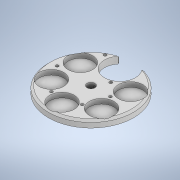
# Autodesk Inventor part: carousel_print
Saved by Autodesk Inventor 2021 (Build 250183000, 183)
## iProperties
Created: 2024-02-22
Part Number: carousel_print
Material: Generic
Document SubType Name: Modeling
Designer: Sebastián
Density: 1 g/cm^3
Appearance: Default
Author: Sebastián
Autodesk Inventor part; units mm, degrees
ref_plane "YZ Plane" through (0, 0, 0) normal (1, 0, 0) x (0, 1, 0)
ref_plane "XZ Plane" through (0, 0, 0) normal (0, 1, 0) x (-1, 0, 0)
ref_plane "XY Plane" through (0, 0, 0) normal (0, 0, 1) x (1, 0, 0)
sketch "Sketch1" plane through (0, 0, 0) normal (0, 1, 0) x (-1, 0, 0)
  circle A0 centre (0, 0) radius 44 construction
  circle A1 centre (0, 0) radius 4.1
  line L0 (0, -30) -> (-25.9808, -15) construction
  line L1 (-25.9808, -15) -> (-25.9808, 15) construction
  line L2 (-25.9808, 15) -> (0, 30) construction
  line L3 (0, 30) -> (25.9808, 15) construction
  line L4 (25.9808, 15) -> (25.9808, -15) construction
  line L5 (25.9808, -15) -> (0, -30) construction
  circle A2 centre (0, -30) radius 12.7 construction
  circle A3 centre (0, -30) radius 16 construction
  circle A4 centre (25.9808, -15) radius 12.7 construction
  arc A5 (9.3274, -43) -> (-9.3274, -43) centre (0, -30) ccw construction
  arc A6 (9.3274, -43) -> (-9.3274, -43) centre (0, 0) ccw
  line L6 (0, -64) -> (0, 62) projected
  arc A7 (9.3274, -43) -> (-9.3274, -43) centre (0, -30) ccw
  dimension "d0" = 88
  dimension "d4" = 32
  dimension "d1" = 8.2
  dimension "d2" = 25.4
  dimension "d3" = 30
  dimension "d5" = 25.4
  constraints: 12 end point, 9 coincident, 6 centre point, 6 point on circle, 1 point on line, 19 other
  measures "d1" diameter of A1
  measures "d2" diameter of A2
  measures "d3" distance of L0.start point (0, 0)
  measures "d5" diameter of A4
extrude "Extrusion1" add sketch "Sketch1" along normal blind 7 contours A1 L6 A6 A7 | A1 L6 A7 A6
sketch "Sketch2" plane through (0, 7, 0) normal (0, 1, 0) x (1, 0, 0)
  arc A0 (-9.3274, 43) -> (9.3274, 43) centre (0, 30) ccw construction
  line L0 (0, 30) -> (25.9808, 15) construction
  line L1 (25.9808, 15) -> (25.9808, -15) construction
  line L2 (25.9808, -15) -> (0, -30) construction
  line L3 (0, -30) -> (-25.9808, -15) construction
  line L4 (-25.9808, -15) -> (-25.9808, 15) construction
  line L5 (-25.9808, 15) -> (0, 30) construction
  circle A1 centre (-25.9808, 15) radius 12.7
  circle A2 centre (-25.9808, -15) radius 12.7
  circle A3 centre (0, -30) radius 12.7
  circle A4 centre (25.9808, -15) radius 12.7
  circle A5 centre (25.9808, 15) radius 12.7
  point P0 (0, 0)
  point P1 (0, 0)
  dimension "d8" = 25.4
  constraints: 12 end point, 6 coincident, 5 centre point, 4 equal radius, 13 other
  measures "d8" diameter of A1
extrude "Extrusion2" cut sketch "Sketch2" against normal blind 5
chamfer "Chamfer1" distance 2 angle 45 1 edges at (0, 7, 44)
chamfer "Chamfer2" distance 4 angle 45 2 edges at (-9.3274, 2.5, -43) (9.3274, 2.5, -43)
sketch "Sketch3" plane through (0, 0, 0) normal (0, 0, 1) x (1, 0, 0)
  circle A0 centre (0, 3.5) radius 1.35
  line L0 (-16, 0) -> (16, 0) projected
  point P0 (0, 0)
  point P1 (12.2604, 0)
  point P2 (-12.2604, 0)
  dimension "d17" = 3.5
  dimension "d18" = 2.7
  constraints: 1 centre point
  measures "d17" distance from line of L0 A0.centre
  measures "d18" diameter of A0
extrude "Extrusion3" cut sketch "Sketch3" against normal through all
sketch "Sketch4" plane through (0, 7, 0) normal (0, 1, 0) x (1, 0, 0)
  circle A0 centre (-25.9808, 15) radius 12.7 construction
  arc A1 (-33.6678, -25.1094) -> (-38.5793, -16.6024) centre (-25.9808, -15) ccw construction
  arc A2 (4.9115, -41.7118) -> (-4.9115, -41.7118) centre (0, -30) ccw construction
  arc A3 (38.5793, -16.6024) -> (33.6678, -25.1094) centre (25.9808, -15) ccw construction
  arc A4 (33.6678, 25.1094) -> (38.5793, 16.6024) centre (25.9808, 15) ccw construction
  circle A5 centre (0, 0) radius 4.1 construction
  line L0 (0, 0) -> (0, -30) construction
  circle A6 centre (0, 0) radius 40 construction
  circle A7 centre (0, 0) radius 35 construction
  circle A8 centre (0, 0) radius 30 construction
  circle A9 centre (0, 0) radius 25 construction
  circle A10 centre (0, 0) radius 20 construction
  circle A11 centre (0, 0) radius 15 construction
  line L1 (61.6, 0) -> (-61.6, 0) construction
  circle A12 centre (7.5, 12.9904) radius 1.5
  circle A13 centre (-20, 34.641) radius 1.5
  circle A14 centre (-35, 0) radius 1.5
  circle A15 centre (-15, -25.9808) radius 1.5
  circle A16 centre (12.5, -21.6506) radius 1.5
  circle A17 centre (20, 0) radius 1.5
  line L2 (0, 59.1703) -> (0, -61.195) construction
  dimension "d28" = 80
  dimension "d29" = 70
  dimension "d30" = 60
  dimension "d31" = 50
  dimension "d32" = 40
  dimension "d38" = 30
  dimension "d45" = 3
  dimension "d46" = 60
  dimension "d47" = 60
  dimension "d48" = 60
  dimension "d49" = 60
  constraints: 6 centre point, 6 coincident, 5 equal radius, 2 end point, 2 horizontal alignment, 2 point on line, 1 vertical, 16 other
  measures "d45" diameter of A12
extrude "Extrusion4" cut sketch "Sketch4" against normal through all
body "Solid1"
